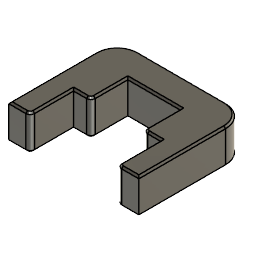
MGN12_rail_guide_x2 (Autodesk Fusion 360 design; units mm, degrees)
part number: 2026-06-27-11-29-30-532
Autodesk Fusion 360 part; units mm, degrees
other "Base Mesh Feature1"
sketch "Sketch1" plane through (0, 0, 0) normal (0, 0, 1) x (1, 0, 0)
  line L0 (0, 6) -> (0, 12.5)
  line L1 (-15, -12.5) -> (-15, 12.5)
  line L2 (-15, 12.5) -> (0, 12.5)
  line L3 (-15, -12.5) -> (-10.05, -12.5)
  line L4 (-10.05, -12.5) -> (-10.05, -2.5)
  line L5 (-10.05, -2.5) -> (-6.05, -2.5)
  line L6 (-6.05, -2.5) -> (-6.05, 6)
  line L7 (-6.05, 6) -> (0, 6)
  dimension "d2" = 15
  dimension "d4" = 6.05
  dimension "d5" = 10.05
  dimension "d6" = 12.5
  dimension "d7" = 6.5
  dimension "d8" = 15
  dimension "d9" = 25
  constraint vertical L0
  constraint parallel L0 L1
  constraint perpendicular L1 L2
  constraint perpendicular L1 L3
  constraint perpendicular L3 L4
  constraint perpendicular L4 L5
  constraint perpendicular L5 L6
  constraint perpendicular L0 L7
  measures "d2" distance of L0 L1
  measures "d4" distance of L0 L6
  measures "d5" distance of L0 L4
  measures "d6" distance of origin L2
  measures "d7" distance of L2 L7
  measures "d8" distance of L2 L5
  measures "d9" distance of L2 L3
extrude "Extrude1" add sketch "Sketch1" along normal blind 8
mirror "Mirror1" about plane through (0, 0, 0) normal (1, 0, 0) of bodies 1 merged
fillet "Fillet1" radius 5 2 edges at (-15, 12.5, 4) (15, 12.5, 4)
fillet "Fillet1" radius 1 4 edges at (-6.05, -2.5, 4) (-10.05, -12.5, 4) (6.05, -2.5, 4) (10.05, -12.5, 4)
chamfer "Chamfer1" distance 0.4 angle 45 2 faces at (2.0167, 10.3333, 8) (2.0167, 10.3333, 0)
